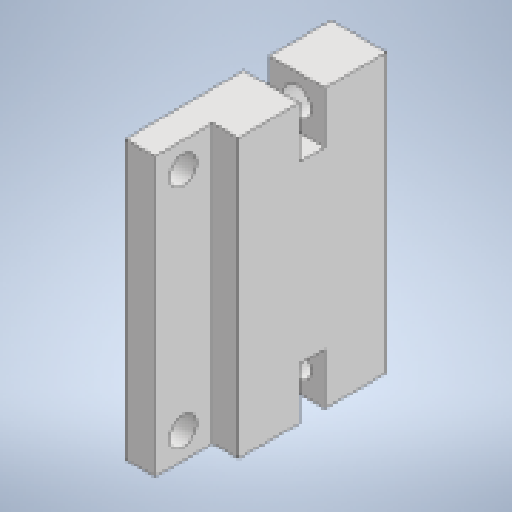
# Autodesk Inventor part: Vertical_Connector_CPY
Saved by Autodesk Inventor 2024.3 (Build 283343000, 343)
## iProperties
Created: 2024-09-06
Part Number: Vertical_Connector_CPY
Material: 일반
Document SubType Name: Modeling
Designer: 구지현
Density: 1 g/cm^3
Appearance: 기본값
Author: 구지현
Autodesk Inventor part; units mm, degrees
ref_plane "YZ Plane" through (0, 0, 0) normal (1, 0, 0) x (0, 1, 0)
ref_plane "XZ Plane" through (0, 0, 0) normal (0, 1, 0) x (-1, 0, 0)
ref_plane "작업 평면1" through (-17.0116, -44.6019, 14.5) normal (0, 0, -1) x (0, 1, 0)
sketch "스케치4" plane through (0, 0, 0) normal (0, 0, 1) x (1, 0, 0)
  arc A0 (-34.0751, 6.2636) -> (-34.5943, 4.5766) centre (-31.5943, 4.5766) ccw projected
  line L0 (-34.5943, -39.6766) -> (-34.5943, 4.5766) projected
  arc A1 (-34.5943, -39.6766) -> (-34.0751, -41.3636) centre (-31.5943, -39.6766) ccw projected
  line L1 (-30.3872, -46.7869) -> (-34.0751, -41.3636) projected
  arc A2 (-30.3872, -46.7869) -> (-27.9064, -48.1) centre (-27.9064, -45.1) ccw projected
  line L2 (-1.0822, -48.1) -> (-27.9064, -48.1) projected
  arc A3 (-1.0822, -48.1) -> (1.3986, -46.7869) centre (-1.0822, -45.1) ccw projected
  line L3 (5.0865, -41.3636) -> (1.3986, -46.7869) projected
  arc A4 (5.0865, -41.3636) -> (5.6057, -39.6766) centre (2.6057, -39.6766) ccw projected
  line L4 (5.6057, 4.5766) -> (5.6057, -39.6766) projected
  arc A5 (5.6057, 4.5766) -> (5.0865, 6.2636) centre (2.6057, 4.5766) ccw projected
  line L5 (1.1009, 12.1246) -> (5.0865, 6.2636) projected
  arc A6 (1.1009, 12.1246) -> (-0.5529, 13) centre (-0.5529, 11) ccw projected
  line L6 (-6.8443, 13) -> (-0.5529, 13) projected
  arc A7 (-5.3443, 11.5) -> (-6.8443, 13) centre (-6.8443, 11.5) ccw projected
  line L7 (-5.3443, 11.5) -> (-5.3443, 10) projected
  arc A8 (-5.3443, 10) -> (-2.9943, 7.65) centre (-2.9943, 10) ccw projected
  line L8 (-2.9943, 7.65) -> (-0.9943, 7.65) projected
  arc A9 (0.0057, 6.65) -> (-0.9943, 7.65) centre (-0.9943, 6.65) ccw projected
  line L9 (0.0057, 6.65) -> (0.0057, -36.15) projected
  arc A10 (-0.9943, -37.15) -> (0.0057, -36.15) centre (-0.9943, -36.15) ccw projected
  line L10 (-0.9943, -37.15) -> (-2.9943, -37.15) projected
  arc A11 (-2.9943, -37.15) -> (-5.3443, -39.5) centre (-2.9943, -39.5) ccw projected
  line L11 (-5.3443, -39.5) -> (-5.3443, -41.5) projected
  arc A12 (-6.3443, -42.5) -> (-5.3443, -41.5) centre (-6.3443, -41.5) ccw projected
  line L12 (-6.3443, -42.5) -> (-22.6443, -42.5) projected
  arc A13 (-23.6443, -41.5) -> (-22.6443, -42.5) centre (-22.6443, -41.5) ccw projected
  line L13 (-23.6443, -41.5) -> (-23.6443, -39.5) projected
  arc A14 (-23.6443, -39.5) -> (-25.9943, -37.15) centre (-25.9943, -39.5) ccw projected
  line L14 (-25.9943, -37.15) -> (-27.9943, -37.15) projected
  arc A15 (-28.9943, -36.15) -> (-27.9943, -37.15) centre (-27.9943, -36.15) ccw projected
  line L15 (-28.9943, -36.15) -> (-28.9943, 6.65) projected
  arc A16 (-27.9943, 7.65) -> (-28.9943, 6.65) centre (-27.9943, 6.65) ccw projected
  line L16 (-27.9943, 7.65) -> (-25.9943, 7.65) projected
  arc A17 (-25.9943, 7.65) -> (-23.6443, 10) centre (-25.9943, 10) ccw projected
  line L17 (-23.6443, 10) -> (-23.6443, 11.5) projected
  arc A18 (-22.1443, 13) -> (-23.6443, 11.5) centre (-22.1443, 11.5) ccw projected
  line L18 (-28.4357, 13) -> (-22.1443, 13) projected
  arc A19 (-28.4357, 13) -> (-30.0896, 12.1246) centre (-28.4357, 11) ccw projected
  line L19 (-34.0751, 6.2636) -> (-30.0896, 12.1246) projected
  circle A20 centre (2.8057, 4) radius 1.35 projected
  circle A21 centre (2.8057, -18) radius 1.35 projected
  circle A22 centre (-3.4943, -45.3) radius 1.35 projected
  circle A23 centre (-31.7943, 4) radius 1.35 projected
  circle A24 centre (-31.7943, -18) radius 1.35 projected
  circle A25 centre (-25.4943, -45.3) radius 1.35 projected
  circle A26 centre (2.8057, -40) radius 1.35 projected
  circle A27 centre (-31.7943, -40) radius 1.35 projected
  line L20 (-31.7943, -40) -> (-31.7943, -18)
  line L21 (-29.0943, -15.5) -> (-34.4943, -15.5)
  line L22 (-34.4943, -15.5) -> (-34.4943, -42.5)
  line L23 (-34.4943, -42.5) -> (-29.0943, -42.5)
  line L24 (-29.0943, -42.5) -> (-29.0943, -15.5)
  line L25 (-29.0943, -15.5) -> (-34.4943, -42.5) construction
  line L26 (-34.4943, -15.5) -> (-29.0943, -42.5) construction
  point P0 (0, 0)
  point P1 (-31.7943, -29)
  dimension "d10" = 5.4
  dimension "d11" = 27
  constraints: 14 end point, 3 midpoint, 2 parallel, 1 horizontal, 1 perpendicular, 1 vertical
  measures "d10" distance of L23.end L22.end
  measures "d11" distance of L22.end L21.end
extrude "돌출4" add sketch "스케치4" against normal blind 6 contours L22 L21 L24 L23 L1 A1 | A1 L1 L23 L22
sketch "스케치5" plane through (0, 0, 0) normal (0, 0, 1) x (1, 0, 0)
  line L0 (-34.4943, -15.5) -> (-34.4943, -42.5) projected
  line L1 (-34.4943, -42.5) -> (-29.0943, -42.5) projected
  line L2 (-29.0943, -42.5) -> (-29.0943, -15.5) projected
  line L3 (-29.0943, -15.5) -> (-34.4943, -15.5) projected
  circle A0 centre (-31.7943, -40) radius 1.35 projected
  circle A1 centre (-31.7943, -18) radius 1.35 projected
  point P0 (0, 0)
extrude "돌출5" add sketch "스케치5" along normal blind 14.4 contours L3 L2 L1 L0 | A0 | A1
sketch "스케치6" plane through (-34.4943, -42.5, -6) normal (-1, 0, 0) x (0, 0, 1)
  line L0 (25.6, 57) -> (29.1, 57)
  line L1 (25.6, 57) -> (20.5, 51)
  line L2 (20.5, 51) -> (20.5, -2.1)
  line L3 (20.5, -2.1) -> (25.6, -8.1)
  line L4 (25.6, -8.1) -> (55.6, -8.1)
  line L5 (55.6, -8.1) -> (60.7, -2.1)
  line L6 (60.7, -2.1) -> (60.7, 51)
  line L7 (60.7, 51) -> (55.6, 57)
  line L8 (52.1, 57) -> (55.6, 57)
  arc A0 (55.1, 54) -> (52.1, 57) centre (52.1, 54) ccw
  line L9 (55.1, 0.5) -> (55.1, 54)
  arc A1 (52.1, -2.5) -> (55.1, 0.5) centre (52.1, 0.5) ccw
  line L10 (29.1, -2.5) -> (52.1, -2.5)
  arc A2 (26.1, 0.5) -> (29.1, -2.5) centre (29.1, 0.5) ccw
  line L11 (26.1, 54) -> (26.1, 0.5)
  arc A3 (29.1, 57) -> (26.1, 54) centre (29.1, 54) ccw
  circle A4 centre (57.9, 46.5) radius 1.35
  circle A5 centre (57.9, 24.5) radius 1.35
  circle A6 centre (57.9, 2.5) radius 1.35
  circle A7 centre (51.6, -5.3) radius 1.35
  circle A8 centre (23.3, 46.5) radius 1.35
  circle A9 centre (23.3, 24.5) radius 1.35
  circle A10 centre (23.3, 2.5) radius 1.35
  circle A11 centre (29.6, -5.3) radius 1.35
  line L12 (20.4, 27) -> (0, 27)
  line L13 (0, 0) -> (0, 27)
  line L14 (0, 0) -> (20.4, 0)
  line L15 (20.4, 27) -> (20.4, 0)
  line L16 (20.4, 0) -> (20.4, 27)
  line L17 (20.4, 27) -> (26, 27)
  line L18 (26, 27) -> (26, 0)
  line L19 (26, 0) -> (20.4, 0)
  line L20 (25.6959, -1.4327) -> (25.7781, -6.0132)
  line L21 (68.9946, 18.9724) -> (67.812, 18.9512)
  arc A12 (65.7765, 20.915) -> (67.812, 18.9512) centre (67.7762, 20.9508) ccw
  line L22 (65.7765, 20.915) -> (65.7397, 22.9646)
  arc A13 (65.7397, 22.9646) -> (64.7219, 23.9465) centre (64.7399, 22.9467) ccw
  line L23 (64.7219, 23.9465) -> (31.7272, 23.3545)
  arc A14 (31.7272, 23.3545) -> (30.7453, 22.3368) centre (31.7452, 22.3547) ccw
  line L24 (30.7453, 22.3368) -> (30.7821, 20.2871)
  arc A15 (28.8183, 18.2515) -> (30.7821, 20.2871) centre (28.7824, 20.2512) ccw
  line L25 (28.8183, 18.2515) -> (26.8186, 18.2157)
  arc A16 (26.8186, 18.2157) -> (25.8367, 17.1979) centre (26.8366, 17.2158) ccw
  line L26 (25.8367, 17.1979) -> (26.0574, 4.8999)
  arc A17 (26.0574, 4.8999) -> (27.0752, 3.918) centre (27.0572, 4.9178) ccw
  line L27 (27.0752, 3.918) -> (29.0748, 3.9538)
  arc A18 (31.1104, 1.99) -> (29.0748, 3.9538) centre (29.1107, 1.9542) ccw
  line L28 (31.1104, 1.99) -> (31.1472, -0.0596)
  arc A19 (31.1472, -0.0596) -> (32.165, -1.0415) centre (32.147, -0.0417) ccw
  line L29 (32.165, -1.0415) -> (65.1596, -0.4495)
  arc A20 (65.1596, -0.4495) -> (66.1415, 0.5682) centre (65.1417, 0.5503) ccw
  line L30 (66.1415, 0.5682) -> (66.1048, 2.6179)
  arc A21 (68.0686, 4.6535) -> (66.1048, 2.6179) centre (68.1044, 2.6538) ccw
  line L31 (68.0686, 4.6535) -> (69.2511, 4.6747)
  spline S0 degree 3 poles (69.2511, 4.6747) (69.5339, 4.6798) (69.869, 4.7337) (70.3387, 4.9133) (70.5662, 5.0474) (70.8526, 5.3129) (70.9739, 5.4731) (71.0515, 5.6305) knots 0 0 0 0 0.420045 0.420045 0.746892 0.746892 1 1 1 1
  line L32 (71.1676, -0.8418) -> (71.0515, 5.6305)
  line L33 (65.2601, -6.0486) -> (71.1676, -0.8418)
  line L34 (26.6663, -6.7411) -> (65.2601, -6.0486)
  line L35 (20.5758, -1.7496) -> (26.6663, -6.7411)
  line L36 (20.1201, 23.6464) -> (20.5758, -1.7496)
  line L37 (26.0277, 28.8532) -> (20.1201, 23.6464)
  line L38 (64.6215, 29.5456) -> (26.0277, 28.8532)
  line L39 (70.712, 24.5541) -> (64.6215, 29.5456)
  line L40 (70.8281, 18.0818) -> (70.712, 24.5541)
  spline S1 degree 3 poles (70.8281, 18.0818) (70.7449, 18.2363) (70.6179, 18.3921) (70.3222, 18.6471) (70.09, 18.7729) (69.6142, 18.9356) (69.2774, 18.9775) (68.9946, 18.9724) knots 0 0 0 0 0.253108 0.253108 0.579955 0.579955 1 1 1 1
  circle A22 centre (63.1719, 26.7192) radius 1.35
  circle A23 centre (46.1747, 26.4142) radius 1.35
  circle A24 centre (22.995, 19.4973) radius 1.35
  circle A25 centre (63.7101, -3.276) radius 1.35
  circle A26 centre (46.7129, -3.581) radius 1.35
  circle A27 centre (23.3, 2.5) radius 1.35
  circle A28 centre (29.1774, 26.1092) radius 1.35
  circle A29 centre (29.7156, -3.8859) radius 1.35
  line L41 (26, 23.5159) -> (0, 23.5159)
  point P0 (6, 42.5)
  dimension "d16" = 5.6
  constraints: 10 end point, 3 parallel, 2 point on line, 1 horizontal, 1 perpendicular
  measures "d16" distance of L12.start L17.end
extrude "돌출6" add sketch "스케치6" against normal blind 2.9 contours L17 L37 L2 | L2 L37 L15 L17 | L37 L17 L18 L41 A9 L2 | L2 L41 L15 L37 | L41 A9 L18 A16 L26 L19 L36 L2 | L2 L36 L15 L41 | L18 L26 A16 | L36 L19 L2 | L2 L19 L15 L36 | A24
sketch "스케치7" plane through (-34.4943, -42.5, -6) normal (-1, 0, 0) x (0, 0, 1)
  line L0 (0, 1.15) -> (0, 3.85) projected
  line L1 (6, 3.85) -> (6, 1.15) projected
  line L2 (0, 23.15) -> (0, 25.85) projected
  line L3 (0, 23.15) -> (0, 25.85) projected
  line L4 (6, 2.5) -> (0, 2.5)
  line L5 (0, 2.5) -> (0, 24.5)
  line L6 (0, 24.5) -> (6, 24.5)
  line L7 (6, 24.5) -> (6, 2.5)
  line L8 (6, 2.5) -> (6, 24.5)
  line L9 (6, 24.5) -> (7.25, 24.5)
  line L10 (7.25, 24.5) -> (7.25, 2.5)
  line L11 (7.25, 2.5) -> (6, 2.5)
  line L12 (8.5, 5) -> (6, 5)
  line L13 (6, 5) -> (6, 0)
  line L14 (6, 0) -> (8.5, 0)
  line L15 (8.5, 0) -> (8.5, 5)
  line L16 (8.5, 5) -> (6, 0) construction
  line L17 (6, 5) -> (8.5, 0) construction
  line L18 (8.5, 22) -> (6, 22)
  line L19 (6, 22) -> (6, 27)
  line L20 (6, 27) -> (8.5, 27)
  line L21 (8.5, 27) -> (8.5, 22)
  line L22 (8.5, 22) -> (6, 27) construction
  line L23 (6, 22) -> (8.5, 27) construction
  point P0 (6, 42.5)
  point P1 (6, 5)
  point P2 (6, 1.15)
  dimension "d19" = 1.25
  dimension "d20" = 2.5
  dimension "d21" = 5
  dimension "d22" = 2.5
  dimension "d23" = 5
  constraints: 40 end point, 8 parallel, 6 midpoint, 5 perpendicular, 3 horizontal
  measures "d19" distance of L6.end L9.end
  measures "d20" distance of L14.end L13.end
  measures "d21" distance of L13.end L12.end
  measures "d22" distance of L19.end L20.end
  measures "d23" distance of L18.end L19.end
extrude "돌출7" cut sketch "스케치7" against normal through all contours L11 L10 L12 L15 L14 L13 L1 | L1 L7 L12 L10 L11 | L9 L10 L18 L7 | L19 L20 L21 L18 L10 L9
move faces "이동1" translate (0, 0, 6) faces at (-29.5959, -25.5425, -6) (-32.6943, -37.5, 1.6667) (-32.6943, -20.5, 0.8333) (-30.8943, -17.1667, 2.5) (-29.5443, -18, 0) (-30.4487, -18.1086, -4) (-30.8943, -15.5, -2) (-30.8943, -39.1667, 2.5) (-29.5443, -40, 0) (-30.4487, -40.1086, -4) (-32.6943, -42.5, -4)
